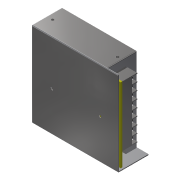
# Autodesk Inventor part: RQ-50B
Saved by Autodesk Inventor 2022 (Build 260153000, 153)
## iProperties
Created: 2015-03-13
Part Number: RQ-50B
Material: Сталь, легированная
Document SubType Name: Modeling
Designer: Oleg
Mass: 2405.47 g
Surface Area: 359.26 cm^2
Volume: 306.429 cm^3
Density: 7.85 g/cm^3
Appearance: С умеренной полировкой
Author: Oleg
Autodesk Inventor part; units mm, degrees
ref_plane "YZ Plane" through (0, 0, 0) normal (1, 0, 0) x (0, 1, 0)
ref_plane "XZ Plane" through (0, 0, 0) normal (0, 1, 0) x (-1, 0, 0)
sketch "Эскиз1" plane through (0, 0, 0) normal (0, 1, 0) x (-1, 0, 0)
  line L0 (-49.5, 48.5) -> (49.5, 48.5)
  line L1 (49.5, 48.5) -> (49.5, -48.5)
  line L2 (49.5, -48.5) -> (-49.5, -48.5)
  line L3 (-49.5, -48.5) -> (-49.5, 48.5)
  line L4 (49.5, 48.5) -> (-49.5, -48.5) construction
  circle A0 centre (29, -3) radius 1.5
  circle A1 centre (-26.5, -3) radius 1.5
  point P0 (0, 0)
  point P1 (0, 0)
  dimension "d0" = 99
  dimension "d1" = 97
  dimension "d15" = 55.5
  dimension "d16" = 20.5
  dimension "d17" = 3
  dimension "d18" = 51.5
  dimension "d19" = 51.5
  constraints: 10 end point, 2 centre point, 2 parallel, 1 coincident, 1 equal radius, 1 horizontal, 1 midpoint, 1 perpendicular
  measures "d0" distance of L1.end L2.end
  measures "d1" distance of L1.end L0.end
  measures "d15" distance of A1.centre A0.centre
  measures "d16" distance from line of L1 A0.centre
  measures "d17" diameter of A1
  measures "d18" distance from line of L0 A1.centre
  measures "d19" distance from line of L0 A0.centre
extrude "Выдавливание1" add sketch "Эскиз1" along normal blind 35 contours L0 L1 L2 L3 | A0 | A1
sketch "Эскиз2" plane through (0, 35, 0) normal (0, 1, 0) x (1, 0, 0)
  line L0 (49.5, -48.5) -> (49.5, 48.5) projected
  line L1 (49.5, 48.5) -> (-49.5, 48.5) projected
  line L2 (49.5, -48.5) -> (36.5, -48.5)
  line L3 (36.5, -48.5) -> (36.5, 47.5)
  line L4 (36.5, 47.5) -> (49.5, 47.5)
  line L5 (49.5, 47.5) -> (49.5, -48.5)
  point P0 (0, 0)
  dimension "d4" = 1
  dimension "d5" = 13
  constraints: 8 end point, 2 parallel, 1 horizontal, 1 perpendicular
  measures "d4" distance between parallel lines of L1 L4
  measures "d5" distance between parallel lines of L0 L3
extrude "Выдавливание2" cut sketch "Эскиз2" against normal blind 34
sketch "Эскиз3" plane through (0, 1, 0) normal (0, 1, 0) x (1, 0, 0)
  line L0 (49.5, 47.5) -> (49.5, -48.5) projected
  line L1 (36.5, -48.5) -> (36.5, 47.5) projected
  line L2 (49.5, -48.5) -> (36.5, -48.5) projected
  line L3 (38.5, 28.5) -> (49.5, 28.5)
  line L4 (49.5, 28.5) -> (49.5, -38.5)
  line L5 (49.5, -38.5) -> (38.5, -38.5)
  line L6 (38.5, -38.5) -> (38.5, 28.5)
  point P0 (0, 0)
  dimension "d8" = 67
  dimension "d9" = 10
  dimension "d10" = 2
  constraints: 8 end point, 2 parallel, 1 horizontal, 1 perpendicular, 1 point on line
  measures "d8" distance of L5.end L3.start
  measures "d9" distance between parallel lines of L2 L5
  measures "d10" distance between parallel lines of L1 L6
extrude "Выдавливание3" add sketch "Эскиз3" along normal blind 15
sketch "Эскиз5" plane through (0, 0, 0) normal (0, -1, 0) x (1, 0, 0)
  line L0 (-49.5, -48.5) -> (49.5, -48.5) projected
  line L1 (49.5, -48.5) -> (49.5, 48.5) projected
  circle A0 centre (29, -3) radius 1.3416
  circle A1 centre (-26, -3) radius 1.5
  point P0 (0, 0)
  dimension "d20" = 3
  dimension "d21" = 45.5
  dimension "d22" = 45.5
  dimension "d23" = 55
  dimension "d24" = 20.5
  constraints: 2 centre point
  measures "d20" diameter of A1
  measures "d21" distance from line of L0 A1.centre
  measures "d22" distance from line of L0 A0.centre
  measures "d23" distance of A0.centre A1.centre
  measures "d24" distance from line of L1 A0.centre
extrude "Выдавливание5" cut sketch "Эскиз5" against normal through all
sketch "Эскиз8" plane through (49.5, 0, -48.5) normal (0, 0, -1) x (-1, 0, 0)
  circle A0 centre (18, 17.5) radius 1.5
  line L0 (0, 35) -> (99, 35) projected
  line L1 (0, 0) -> (0, 35) projected
  circle A1 centre (92, 17.1646) radius 1.5
  point P0 (49.5, 0)
  dimension "d43" = 3
  dimension "d44" = 74
  dimension "d45" = 18
  dimension "d46" = 17.5
  constraints: 2 centre point, 1 equal radius
  measures "d43" diameter of A1
  measures "d44" horizontal distance of A1.centre A0.centre
  measures "d45" distance from line of L1 A0.centre
  measures "d46" distance from line of L0 A0.centre
extrude "Выдавливание10" cut sketch "Эскиз8" against normal through all
sketch "Эскиз9" plane through (38.5, 1, 38.5) normal (0, 0, 1) x (1, 0, 0)
  line L0 (11, 0) -> (0, 0)
  line L1 (0, 0) -> (0, 21)
  line L2 (0, 21) -> (11, 21)
  line L3 (11, 21) -> (11, 0)
  point P0 (-38.5, -1)
  dimension "d47" = 21
  constraints: 8 end point, 2 parallel, 1 horizontal, 1 perpendicular
  measures "d47" distance of L2.end L0.start
extrude "Выдавливание11" add sketch "Эскиз9" along normal blind 1
pattern_linear "Прямоуг.массив1" count 9 spacing 8.5 along (0, 0, -1) of "Выдавливание11"
sketch "Эскиз10" plane through (0, 16, 0) normal (0, 1, 0) x (1, 0, 0)
  line L0 (49.5, -38.5) -> (49.5, -31) projected
  line L1 (38.5, -31) -> (49.5, -38.5) construction
  line L2 (49.5, -31) -> (38.5, -38.5) construction
  circle A0 centre (44, -34.75) radius 3.5
  circle A1 centre (44, -26.25) radius 3.5
  circle A2 centre (44, -17.75) radius 3.5
  circle A3 centre (44, -9.25) radius 3.5
  circle A4 centre (44, -0.75) radius 3.5
  circle A5 centre (44, 7.75) radius 3.5
  circle A6 centre (44, 16.25) radius 3.5
  circle A7 centre (44, 24.75) radius 3.5
  point P0 (0, 0)
  dimension "d53" = 7
  dimension "d56" = 8.5
  constraints: 8 centre point, 4 end point, 1 midpoint, 1 vertical, 14 other
  measures "d53" diameter of A0
  measures "d56" distance of A0.centre A1.centre
extrude "Выдавливание12" add sketch "Эскиз10" along normal blind 4
fillet "Сопряжение1" radius 1 8 edges at (40.5, 20, 34.75) (40.5, 20, 26.25) (40.5, 20, 17.75) (40.5, 20, 9.25) (40.5, 20, 0.75) (40.5, 20, -7.75) (40.5, 20, -16.25) (40.5, 20, -24.75)
sketch "Эскиз11" plane through (44, 20, 34.75) normal (0, 1, 0) x (1, 0, 0)
  circle A0 centre (0, 0) radius 2.5 projected
  line L0 (2.3846, 0.7507) -> (2.3846, -0.7507)
  line L1 (-2.381, -0.762) -> (-2.381, 0.762)
  line L2 (-0.8517, 2.3504) -> (0.8517, 2.3504)
  line L3 (0.8327, -2.3572) -> (-0.8327, -2.3572)
  line L4 (-0.8327, -2.3572) -> (-0.8327, -0.762)
  line L5 (-0.8517, 0.762) -> (-0.8517, 2.3504)
  line L6 (-2.381, 0.762) -> (-0.8517, 0.762)
  line L7 (0.8517, 0.7507) -> (2.3846, 0.7507)
  line L8 (0.8517, 2.3504) -> (0.8517, 0.7507)
  line L9 (0.8327, -0.7507) -> (0.8327, -2.3572)
  line L10 (2.3846, -0.7507) -> (0.8327, -0.7507)
  line L11 (-0.8327, -0.762) -> (-2.381, -0.762)
  point P0 (-44, 34.75)
  constraints: 24 end point, 10 parallel, 4 perpendicular, 3 horizontal, 9 other
extrude "Выдавливание13" cut sketch "Эскиз11" against normal blind 2 contours L0 L10 L9 L3 L4 L11 L1 L6 L5 L2 L8 L7
pattern_linear "Прямоуг.массив2" count 8 spacing 8.5 along (0, 0, -1) of "Выдавливание13"
fillet "Сопряжение2" radius 1 4 edges at (36.5, 35, 0.5) (-6.5, 35, 48.5) (36.5, 18, 48.5) (-49.5, 35, 0)
fillet "Сопряжение3" radius 1 3 edges at (-49.2071, 34.7071, -48.5) (-49.5, 17, -48.5) (0.5, 35, -48.5)
fillet "Сопряжение4" radius 1 6 edges at (0.4999, 0, -48.5) (-49.2071, 0, -48.2071) (-49.5, 0, 0.4999) (0, 0, 48.5) (-49.2071, 34.7071, 48.2071) (-49.5, 17, 48.5)
sketch "Эскиз12" plane through (36.5, 1, 47.5) normal (1, 0, 0) x (0, 0, -1)
  line L0 (0, 0) -> (95, 0) projected
  line L1 (95, 33) -> (95, 0) projected
  line L2 (8, 0) -> (8, 21) projected
  line L3 (95, 34) -> (95, 0) projected
  line L4 (8, 21) -> (95, 21)
  point P0 (47.5, -1)
  constraints: 2 end point, 1 perpendicular, 1 point on line
extrude "Выдавливание14" cut sketch "Эскиз12" against normal blind 84
sketch "Эскиз13" plane through (0, 1, 0) normal (0, 1, 0) x (1, 0, 0)
  circle A0 centre (29, 3) radius 1.3416 projected
  line L0 (-47.5, 47.5) -> (49.5, 47.5) projected
  line L1 (-47.5, 47.5) -> (-47.5, -39.5) projected
  line L2 (36.5, -39.5) -> (-47.5, -39.5) projected
  line L3 (36.5, -47.5) -> (36.5, -39.5) projected
  arc A1 (35.5, -48.5) -> (36.5, -47.5) centre (35.5, -47.5) ccw projected
  line L4 (35.5, -48.5) -> (49.5, -48.5) projected
  line L5 (49.5, -39.5) -> (49.5, -48.5) projected
  line L6 (49.5, -39.5) -> (38.5, -39.5) projected
  line L7 (38.5, -39.5) -> (38.5, 29.5) projected
  line L8 (38.5, 29.5) -> (38.5, 47.5)
  point P0 (0, 0)
  point P1 (-49.5, 47.5)
  point P2 (-49.5, -39.5)
  constraints: 2 end point, 1 collinear, 1 point on line
extrude "Выдавливание15" add sketch "Эскиз13" along normal blind 0.001
sketch "Эскиз15" plane through (0, 1.001, 0) normal (0, 1, 0) x (1, 0, 0)
  line L0 (36.5, -47.5) -> (36.5, -39.5) projected
  line L1 (35.5, -48.5) -> (49.5, -48.5) projected
  line L2 (49.5, -48.5) -> (49.5, -39.5) projected
  line L3 (36.5, -39.5) -> (49.5, -39.5)
  line L4 (49.5, -39.5) -> (49.5, -48.5)
  line L5 (49.5, -48.5) -> (36.5, -48.5)
  line L6 (36.5, -48.5) -> (36.5, -39.5)
  line L7 (49.4, -48.4) -> (36.6, -48.4)
  line L8 (36.6, -48.4) -> (36.6, -39.6)
  line L9 (36.6, -39.6) -> (49.4, -39.6)
  line L10 (49.4, -39.6) -> (49.4, -48.4)
  point P0 (0, 0)
  dimension "d76" = 0.1
  dimension "d77" = 0.1
  dimension "d78" = 0.1
  dimension "d79" = 0.1
  constraints: 16 end point, 4 parallel, 2 horizontal, 2 perpendicular
  measures "d76" distance between parallel lines of L1 L7
  measures "d77" distance between parallel lines of L3 L9
  measures "d78" distance between parallel lines of L2 L10
  measures "d79" distance between parallel lines of L0 L8
extrude "Выдавливание16" add sketch "Эскиз15" along normal blind 0.001 contours L7 L8 L9 L10
ref_plane "Work Plane1" through (0, 3.001, 0) normal (0, 1, 0) x (1, 0, 0)
sketch "Sketch17" plane through (0, 3.001, 0) normal (0, 1, 0) x (1, 0, 0)
  line L0 (36.5, -39.5) -> (36.5, 47.5) projected
  line L1 (36.5, 45.5319) -> (-45.9899, 45.5319)
  line L2 (-45.9899, 45.5319) -> (-45.9899, -45.1394)
  line L3 (-45.9899, -45.1394) -> (36.5, -45.1394)
  line L4 (36.5, -45.1394) -> (36.5, 45.5319)
  point P0 (0, 0)
  constraints: 8 end point, 2 parallel, 1 horizontal, 1 perpendicular, 1 point on line
extrude "Extrusion17" add sketch "Sketch17" along normal blind 2 separate body
sketch "Sketch18" plane through (49.5, 16, 38.5) normal (1, 0, 0) x (0, 0, -1)
  line L0 (-6.6394, -10.999) -> (84.0319, -10.999) projected
  line L1 (69.9569, -10.999) -> (69.9569, -12.999)
  line L2 (-6.6394, -12.999) -> (84.0319, -12.999) projected
  line L3 (-1, 6) -> (-1, -14.999) projected
  line L4 (-1, -10.999) -> (-1, -12.999)
  line L5 (-1, -12.999) -> (69.9569, -12.999)
  point P0 (38.5, -16)
  constraints: 6 end point, 5 point on line, 1 perpendicular, 1 vertical
extrude "Extrusion18" cut sketch "Sketch18" against normal up to surface (13 mm away) bodies 1
sketch "Sketch19" plane through (49.5, 1, -29.5) normal (0, 0, -1) x (-1, 0, 0)
  line L0 (11, 2.001) -> (0, 2.001) projected
  line L1 (0, 0) -> (0, 2.001) projected
  line L2 (11, 0) -> (0, 0) projected
  line L3 (11, 0.001) -> (11, 0) projected
  line L4 (11, 2.001) -> (11, 0.001) projected
  point P0 (49.5, -1)
extrude "Extrusion19" cut sketch "Sketch19" against normal through all bodies 1
sketch "Sketch20" plane through (0, 5.001, 0) normal (0, 1, 0) x (1, 0, 0)
  line L0 (38.5, 47.5) -> (38.5, -39.6) projected
  line L1 (-51.2646, -48.5) -> (38.5, -48.5)
  line L2 (38.5, -48.5) -> (38.5, -39.6)
  line L3 (38.5, -39.6) -> (-51.2646, -39.6)
  line L4 (-51.2646, -39.6) -> (-51.2646, -48.5)
  point P0 (0, 0)
  constraints: 8 end point, 2 parallel, 1 horizontal, 1 perpendicular
extrude "Extrusion20" cut sketch "Sketch20" against normal through all bodies 2
sketch "Sketch22" plane through (36.5, 3.001, -45.5319) normal (1, 0, 0) x (0, 0, -1)
  line L0 (-85.1319, 2) -> (-85.1319, 0) projected
  line L1 (-85.1319, 0) -> (0, 0) projected
  line L2 (0, 0) -> (0, 2) projected
  line L3 (-85.1319, 2) -> (0, 2) projected
  point P0 (-45.5319, -3.001)
extrude "Extrusion21" add sketch "Sketch22" along normal up to surface (13 mm away) bodies 2
sketch "Sketch23" plane through (0, 16, 0) normal (0, 1, 0) x (1, 0, 0)
  circle A0 centre (44, -0.75) radius 3.5 projected
sketch "Sketch24" plane through (0, 16, 0) normal (0, 1, 0) x (1, 0, 0)
  circle A0 centre (44, 7.75) radius 3.5 projected
body "Solid2"
